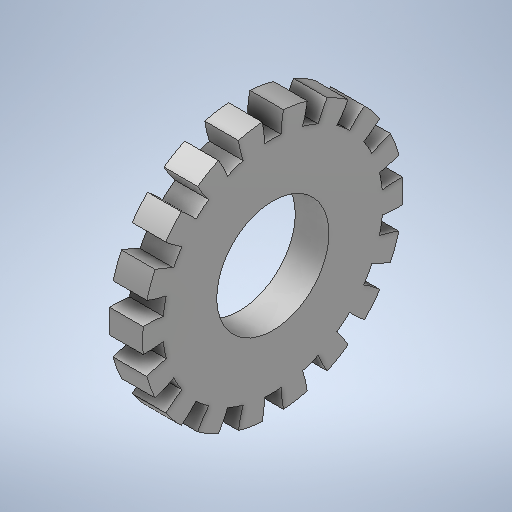
# Autodesk Inventor part: Zahnrad_bei_Laufrad
Saved by Autodesk Inventor 2025.2 (Build 292293000, 293)
## iProperties
Created: 2025-02-03
Part Number: Zahnrad_bei_Laufrad
Material: Generisch
Document SubType Name: Modeling
Designer: unter
Density: 1 g/cm^3
Appearance: Vorgabe
Author: unter
Autodesk Inventor part; units mm, degrees
ref_plane "YZ Plane" through (0, 0, 0) normal (1, 0, 0) x (0, 1, 0)
ref_plane "XZ Plane" through (0, 0, 0) normal (0, 1, 0) x (-1, 0, 0)
ref_plane "XY Plane" through (0, 0, 0) normal (0, 0, 1) x (1, 0, 0)
derived "Skelett_Laufkatze.ipt"
sketch "Zahnrad_Laufrad_seite" plane through (-97, 65, 62.4) normal (0, 0, -1) x (-1, 0, 0)
  line L0 (34, 50) -> (34, 0) construction
  line L1 (34, 25) -> (32, 25) construction
  line L2 (32, 50) -> (32, 83)
  line L3 (32, 83) -> (17, 83)
  line L4 (17, 83) -> (17, 50)
  line L5 (17, 50) -> (32, 50)
  line L6 (32, 25) -> (17, 25)
  point P0 (-97, -65)
sketch "Zahnrad_Laufrad_front" plane through (-129, 115, 62.4) normal (-1, 0, 0) x (0, -1, 0)
  circle A0 centre (25, 0) radius 25
  circle A1 centre (25, 0) radius 58
  circle A2 centre (25, 0) radius 49 construction
  arc A3 (-23.86, -3.7012) -> (-32.8053, -4.7484) centre (-22.456, -54.4252) ccw
  arc A4 (-32.8053, 4.7484) -> (-23.86, 3.7012) centre (-22.456, 54.4252) ccw
  line L0 (25, 0) -> (-33, 0) construction
  arc A5 (-32.8053, 4.7484) -> (-32.8053, -4.7484) centre (25, 0) ccw
  arc A6 (-23.86, 3.7012) -> (-23.86, -3.7012) centre (25, 0) ccw
  circle A7 centre (25, 0) radius 54
  point P0 (115, -62.4)
  point P1 (0, 0)
  point P2 (-24, 0)
revolve "Zahnrad_Rohling" add sketch "Zahnrad_Laufrad_seite" angle 360 about axis through (-129, 90, 62.4) along (1, 0, 0)
extrude "Zahngeometrie" cut sketch "Zahnrad_Laufrad_front" against normal through all contours A4 A7 A3 A1 | A4 A6 A3 A7 picked at (-31.6465, -0.4543) picked at (-27.3167, 0.4116)
pattern_circular "Anzahl_zähne" count 18 over 360 about axis through (-121.5, 90, 62.4) along (1, 0, 0) of "Zahngeometrie"
